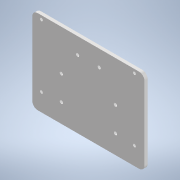
# Autodesk Inventor part: down_plate
Saved by Autodesk Inventor 2020 (Build 240168000, 168)
## iProperties
Created: 2021-05-05
Part Number: down_plate
Material: Типовые
Document SubType Name: Modeling
Designer: tviks
Density: 1 g/cm^3
Appearance: По умолчанию
Author: tviks
Autodesk Inventor part; units mm, degrees
ref_plane "YZ Plane" through (0, 0, 0) normal (1, 0, 0) x (0, 1, 0)
ref_plane "XZ Plane" through (0, 0, 0) normal (0, 1, 0) x (-1, 0, 0)
ref_plane "XY Plane" through (0, 0, 0) normal (0, 0, 1) x (1, 0, 0)
sketch "Эскиз1" plane through (0, 0, 0) normal (0, 0, 1) x (1, 0, 0)
  circle A0 centre (41.8996, -50.8737) radius 1.5 projected
  circle A1 centre (115.8996, -50.8737) radius 1.5 projected
  line L0 (128.2996, -55.7737) -> (128.2996, 12.0263) projected
  arc A2 (128.2996, 12.0263) -> (123.2996, 17.0263) centre (123.2996, 12.0263) ccw projected
  line L1 (123.2996, 17.0263) -> (29.4996, 17.0263) projected
  arc A3 (29.4996, 17.0263) -> (24.4996, 12.0263) centre (29.4996, 12.0263) ccw projected
  line L2 (24.4996, 12.0263) -> (24.4996, -55.7737) projected
  arc A4 (24.4996, -55.7737) -> (29.4996, -60.7737) centre (29.4996, -55.7737) ccw projected
  line L3 (29.4996, -60.7737) -> (123.2996, -60.7737) projected
  arc A5 (123.2996, -60.7737) -> (128.2996, -55.7737) centre (123.2996, -55.7737) ccw projected
  line L4 (53.8996, 12.1263) -> (105.3355, 12.1263) projected
  arc A6 (105.3355, 9.1263) -> (105.3355, 12.1263) centre (105.3355, 10.6263) ccw projected
  line L5 (105.3355, 9.1263) -> (53.8996, 9.1263) projected
  arc A7 (53.8996, 12.1263) -> (53.8996, 9.1263) centre (53.8996, 10.6263) ccw projected
  circle A8 centre (53.8996, -6.8737) radius 1.5 projected
  circle A9 centre (53.8996, -36.8737) radius 1.5 projected
  circle A10 centre (103.8996, -36.8737) radius 1.5 projected
  circle A11 centre (103.8996, -6.8737) radius 1.5 projected
  circle A12 centre (118.8996, -44.3737) radius 1.375 projected
  circle A13 centre (32.8996, -44.3737) radius 1.375 projected
  circle A14 centre (32.8996, 13.6263) radius 1.375 projected
  circle A15 centre (118.8996, 13.6263) radius 1.375 projected
  line L6 (105.3355, -0.8737) -> (53.8996, -0.8737) projected
  arc A16 (53.8996, 2.1263) -> (53.8996, -0.8737) centre (53.8996, 0.6263) ccw projected
  line L7 (53.8996, 2.1263) -> (105.3355, 2.1263) projected
  arc A17 (105.3355, -0.8737) -> (105.3355, 2.1263) centre (105.3355, 0.6263) ccw projected
  arc A18 (53.8996, -42.8737) -> (53.8996, -45.8737) centre (53.8996, -44.3737) ccw projected
  line L8 (53.8996, -42.8737) -> (103.8996, -42.8737) projected
  arc A19 (103.8996, -45.8737) -> (103.8996, -42.8737) centre (103.8996, -44.3737) ccw projected
  line L9 (103.8996, -45.8737) -> (53.8996, -45.8737) projected
  line L10 (103.8996, -55.8737) -> (53.8996, -55.8737) projected
  arc A20 (53.8996, -52.8737) -> (53.8996, -55.8737) centre (53.8996, -54.3737) ccw projected
  line L11 (53.8996, -52.8737) -> (103.8996, -52.8737) projected
  arc A21 (103.8996, -55.8737) -> (103.8996, -52.8737) centre (103.8996, -54.3737) ccw projected
  point P0 (0, 0)
extrude "Выдавливание1" add sketch "Эскиз1" along normal blind 3 contours A0 | A1 | A5 L3 A4 L2 A3 L1 A2 L0 | L4 A6 L5 A7 | A8 | A9 | A10 | A11 | L6 A16 L7 A17 | L8 A19 L9 A18 | L10 A20 L11 A21
sketch "Эскиз2" plane through (0, 0, 3) normal (0, 0, 1) x (1, 0, 0)
  line L0 (29.4996, -60.7737) -> (123.2996, -60.7737) projected
  circle A0 centre (51.3996, -43.2737) radius 1.5
  circle A1 centre (101.3996, -43.2737) radius 1.5
  point P0 (0, 0)
  dimension "d6" = 3
  dimension "d7" = 3
  constraints: 2 centre point
  measures "d6" diameter of A0
  measures "d7" diameter of A1
extrude "Выдавливание2" cut sketch "Эскиз2" against normal blind 3
sketch "Эскиз3" plane through (0, 0, 3) normal (0, 0, 1) x (1, 0, 0)
  line L0 (24.4996, 12.0263) -> (24.4996, -55.7737) projected
  line L1 (24.4996, -21.8737) -> (128.2996, -21.8737)
  line L2 (128.2996, -55.7737) -> (128.2996, 12.0263) projected
  line L3 (76.3996, -21.8737) -> (76.3996, 17.0263)
  line L4 (123.2996, 17.0263) -> (29.4996, 17.0263) projected
  circle A0 centre (118.8996, -44.3737) radius 1.375 projected
  circle A1 centre (101.3996, -43.2737) radius 1.5 projected
  circle A2 centre (51.3996, -20.4987) radius 1.5
  circle A3 centre (101.3996, -20.4987) radius 1.5
  line L5 (76.3996, -20.4987) -> (76.3996, -7.9987)
  line L6 (76.3996, -7.9987) -> (76.3996, 2.0013)
  circle A4 centre (66.3996, 2.0013) radius 1.5
  circle A5 centre (86.3996, 2.0013) radius 1.5
  point P0 (0, 0)
  point P1 (101.999, -21.8737)
  point P2 (100.8001, -21.8737)
  dimension "d13" = 3
  dimension "d14" = 3
  dimension "d19" = 3
  dimension "d20" = 3
  constraints: 8 end point, 4 centre point, 4 midpoint, 2 point on line
  measures "d13" diameter of A2
  measures "d14" diameter of A3
  measures "d19" diameter of A4
  measures "d20" diameter of A5
extrude "Выдавливание3" cut sketch "Эскиз3" against normal blind 3 contours A2 L1 | L1 A2 | A3 L1 | A4 | A5 picked at (100.9144, -20.3462)
